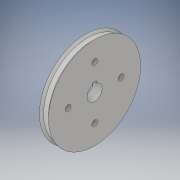
# Autodesk Inventor part: Practica 2 Polea
Saved by Autodesk Inventor 2019.1 (Build 231200000, 200)
## iProperties
Created: 2024-02-06
Part Number: Practica 2 Polea
Material: Generic
Document SubType Name: Modeling
Designer: clariheelen
Density: 1 g/cm^3
Appearance: Default
Author: clariheelen
Autodesk Inventor part; units mm, degrees
ref_plane "YZ Plane" through (0, 0, 0) normal (1, 0, 0) x (0, 1, 0)
ref_plane "XZ Plane" through (0, 0, 0) normal (0, 1, 0) x (-1, 0, 0)
ref_plane "XY Plane" through (0, 0, 0) normal (0, 0, 1) x (1, 0, 0)
sketch "Sketch1" plane through (0, 0, 0) normal (0, 0, 1) x (1, 0, 0)
  line L0 (0, 0) -> (100, 0)
  line L1 (100, 0) -> (100, 500)
  line L2 (0, 500) -> (0, 0)
  line L3 (0, 500) -> (17.6777, 482.3223)
  line L4 (0, 500) -> (25, 500) construction
  line L5 (100, 500) -> (82.3223, 482.3223)
  line L6 (100, 500) -> (125, 500) construction
  line L7 (82.3223, 482.3223) -> (17.6777, 482.3223)
  line L8 (50, -100) -> (-150, -100)
  dimension "d7" = 200
  constraints: 18 end point, 4 horizontal, 2 equal length, 1 parallel, 1 perpendicular
  measures "d7" distance of L8.start L8.end
revolve "Revolution1" add sketch "Sketch1" angle 360 about axis through (50, -100, 0) along (-1, 0, 0)
sketch "Sketch2" plane through (0, -100, 0) normal (-1, 0, 0) x (0, 0, 1)
  circle A0 centre (0, 0) radius 600 projected
  circle A1 centre (350, 0) radius 37.5
  circle A2 centre (0, 0) radius 100
  circle A3 centre (0, -350) radius 37.5
  circle A4 centre (-350, 0) radius 37.5
  circle A5 centre (0, 350) radius 37.5
  point P0 (0, 100)
  dimension "d9" = 75
  dimension "d12" = 360
  constraints: 5 centre point, 1 coincident, 9 other
  measures "d9" diameter of A1
extrude "Extrusion1" cut sketch "Sketch2" against normal blind 200 contours A1 | A3 | A4 | A5
thicken "Thicken1" operation add thickness 10 both sides no extend neighbours yes toward (1, 0, 0) faces at (100, -364.9419, 262.9039)
thicken "Thicken2" operation add thickness 10 both sides no extend neighbours yes toward (-1, 0, 0) faces at (0, -364.9419, 262.9039)
sketch "Sketch3" plane through (-10, -100, 0) normal (-1, 0, 0) x (0, 0, 1)
  line L0 (25, 96.8246) -> (25, 125)
  line L1 (25, 125) -> (-25, 125)
  line L2 (-25, 125) -> (-25, 96.8246)
  line L3 (-25, 75) -> (25, 125) construction
  line L4 (25, 75) -> (-25, 125) construction
  circle A0 centre (0, 0) radius 100 projected
  circle A1 centre (0, 0) radius 100
  point P0 (0, 100)
  constraints: 10 end point, 3 point on circle, 2 midpoint, 1 centre point, 1 coincident, 1 parallel, 1 vertical alignment
extrude "Extrusion2" cut sketch "Sketch3" against normal blind 120 contours A0 L2 L1 L0
body "Solid1"
